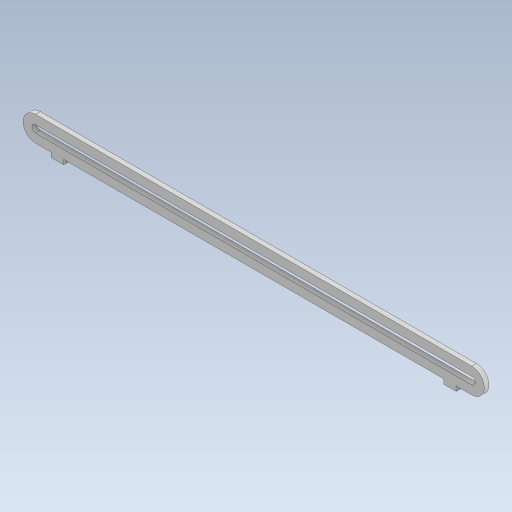
# Autodesk Inventor part: 零件4
Saved by Autodesk Inventor 2023 (Build 270158000, 158)
## iProperties
Created: 2023-04-16
Part Number: 零件4
Material: 一般
Document SubType Name: Modeling
Designer: JOU
Density: 1 g/cm^3
Appearance: 預設
Author: JOU
Autodesk Inventor part; units mm, degrees
ref_plane "YZ Plane" through (0, 0, 0) normal (1, 0, 0) x (0, 1, 0)
ref_plane "XZ Plane" through (0, 0, 0) normal (0, 1, 0) x (-1, 0, 0)
ref_plane "XY Plane" through (0, 0, 0) normal (0, 0, 1) x (1, 0, 0)
sketch "草圖1" plane through (0, 0, 0) normal (0, 0, 1) x (1, 0, 0)
  line L0 (-140, 0) -> (140, 0) construction
  line L1 (-140, 2.3) -> (140, 2.3)
  line L2 (140, -2.3) -> (-140, -2.3)
  arc A0 (-140, 2.3) -> (-140, -2.3) centre (-140, 0) ccw
  arc A1 (140, -2.3) -> (140, 2.3) centre (140, 0) ccw
  line L3 (-140, 0) -> (140, 0) construction
  line L4 (-140, -8) -> (140, -8)
  line L5 (140, 8) -> (-140, 8)
  arc A2 (-140, 8) -> (-140, -8) centre (-140, 0) ccw
  arc A3 (140, -8) -> (140, 8) centre (140, 0) ccw
  point P0 (0, 0)
  point P1 (0, 0)
  point P2 (0, 0)
  dimension "d5" = 8
  dimension "d6" = 2.3
  dimension "d7" = 280
  constraints: 16 end point, 8 point on circle, 8 tangent, 4 centre point, 2 coincident, 2 midpoint, 2 parallel, 2 point on line, 2 vertical alignment, 1 horizontal
  measures "d5" radius of A2
  measures "d6" radius of A0
  measures "d7" distance of L3.end L3.start
extrude "擠出1" add sketch "草圖1" along normal blind 3
sketch "草圖2" plane through (0, 0, 3) normal (0, 0, 1) x (1, 0, 0)
  line L0 (-207.2, 0) -> (207.2, 0) projected
  line L1 (-130, -8) -> (-122, -8)
  line L2 (-122, -8) -> (-122, -11)
  line L3 (-122, -11) -> (-130, -11)
  line L4 (-130, -11) -> (-130, -8)
  line L5 (122, -8) -> (130, -8)
  line L6 (130, -8) -> (130, -11)
  line L7 (130, -11) -> (122, -11)
  line L8 (122, -11) -> (122, -8)
  line L9 (-140, -8) -> (140, -8) projected
  point P0 (0, 0)
  dimension "d16" = 10
  dimension "d17" = 8
  dimension "d18" = 3
  dimension "d19" = 3
  dimension "d20" = 8
  dimension "d21" = 10
  constraints: 16 end point, 5 perpendicular, 2 collinear, 1 parallel
  measures "d16" distance from line of L4 L9.start
  measures "d17" distance of L2.end L3.end
  measures "d18" distance of L1.end L2.end
  measures "d19" distance of L5.end L6.end
  measures "d20" distance of L6.end L7.end
  measures "d21" distance from line of L9.end L6
extrude "擠出2" add sketch "草圖2" against normal up to surface (3 mm away)
